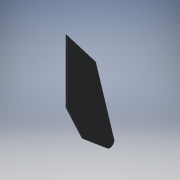
# Autodesk Inventor part: type7_stay
Saved by Autodesk Inventor 2018.1 (Build 221171000, 171)
## iProperties
Created: 2017-11-03
Part Number: type7_stay
Material: CFRP
Document SubType Name: Modeling
Designer: ku_sk
Density: 1.43 g/cm^3
Appearance: カーボンファイバー
Mass: 45.2777 g
Surface Area: 224.647 cm^2
Volume: 31.6627 cm^3
Author: ku_sk
Autodesk Inventor part; units mm, degrees
ref_plane "YZ Plane" through (0, 0, 0) normal (1, 0, 0) x (0, 1, 0)
ref_plane "XZ Plane" through (0, 0, 0) normal (0, 1, 0) x (-1, 0, 0)
ref_plane "XY Plane" through (0, 0, 0) normal (0, 0, 1) x (1, 0, 0)
sketch "スケッチ1" plane through (0, 0, 0) normal (1, 0, 0) x (0, 1, 0)
  line L0 (0, 84.8101) -> (0, -115.1899)
  line L1 (0, -274.6451) -> (0, 144.7193) projected
  line L2 (0, 84.8101) -> (68.0158, -3.9861)
  line L3 (68.0158, -3.9861) -> (118.6619, -214.7359)
  line L4 (118.6619, -214.7359) -> (0, -115.1899)
  point P0 (0, 0)
  dimension "d0" = 200
  constraints: 8 end point, 1 collinear, 1 vertical
  measures "d0" distance of L0.start L0.end
extrude "押し出し1" add sketch "スケッチ1" along normal blind 3
chamfer "面取り1" distance 50 angle 45 1 edges at (1.5, 0, -115.1899)
fillet "フィレット1" radius 10 2 edges at (1.5, 118.6619, -214.7359) (1.5, 68.0158, -3.9861)
